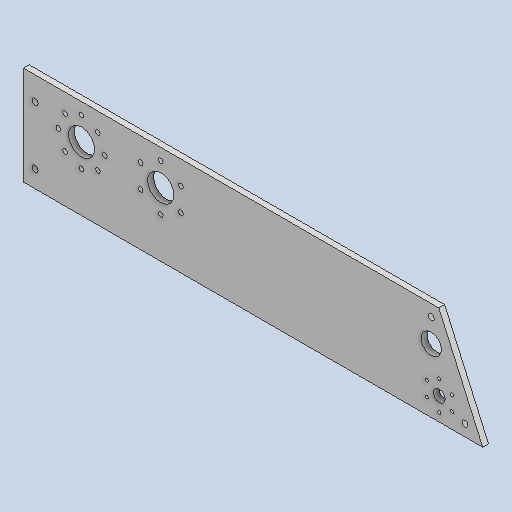
# Autodesk Inventor part: Bottom Part
Saved by Autodesk Inventor 2023 (Build 270158000, 158)
## iProperties
Created: 2023-11-04
Part Number: Bottom Part
Material: Generic
Document SubType Name: Modeling
Designer: jackc
Density: 1 g/cm^3
Appearance: Default
Author: jackc
Autodesk Inventor part; units mm, degrees
ref_plane "YZ Plane" through (0, 0, 0) normal (1, 0, 0) x (0, 1, 0)
ref_plane "XZ Plane" through (0, 0, 0) normal (0, 1, 0) x (-1, 0, 0)
ref_plane "XY Plane" through (0, 0, 0) normal (0, 0, 1) x (1, 0, 0)
sketch "Sketch1" plane through (0, 0, 0) normal (0, 0, 1) x (1, 0, 0)
  circle A0 centre (86.772, 0) radius 50.8 construction
  circle A1 centre (0, 0) radius 29.972 construction
  circle A2 centre (0, 0) radius 25.4 construction
  circle A3 centre (0, 25.4) radius 2.54
  circle A4 centre (17.9605, 17.9605) radius 2.54
  circle A5 centre (-17.9605, 17.9605) radius 2.54
  circle A6 centre (-17.9605, -17.9605) radius 2.54
  circle A7 centre (-25.4, 0) radius 2.54
  circle A8 centre (17.9605, -17.9605) radius 2.54
  circle A9 centre (25.4, 0) radius 2.54
  circle A10 centre (0, -25.4) radius 2.54
  line L0 (0, 25.4) -> (0, 0) construction
  line L1 (0, 0) -> (-17.9605, 17.9605) construction
  circle A11 centre (0, 0) radius 35.972 construction
  line L2 (-63.5, 38.1) -> (-63.5, -69.85)
  line L3 (-63.5, -69.85) -> (438.9497, -69.85)
  circle A12 centre (-50.8, 12.7) radius 3.302
  circle A13 centre (-50.8, -50.8) radius 3.302
  line L4 (-63.5, 38.1) -> (390.9326, 38.1)
  circle A14 centre (86.772, 0) radius 14.2875
  circle A15 centre (0, 0) radius 14.2875
  circle A16 centre (86.772, 0) radius 285.75 construction
  circle A17 centre (382.682, 25.4) radius 3.302
  circle A18 centre (419.4009, -57.15) radius 3.302
  circle A19 centre (86.772, 0) radius 25.4 construction
  circle A20 centre (86.772, 25.4) radius 2.54
  circle A21 centre (64.775, 12.7) radius 2.54
  circle A22 centre (64.775, -12.7) radius 2.54
  circle A23 centre (86.772, -25.4) radius 2.54
  circle A24 centre (108.769, -12.7) radius 2.54
  circle A25 centre (108.769, 12.7) radius 2.54
  circle A26 centre (391.4609, -44.8692) radius 16 construction
  circle A27 centre (391.4609, -44.8692) radius 6.4135
  circle A28 centre (391.4609, -28.8692) radius 1.8
  circle A29 centre (391.4609, -44.8692) radius 22.225 construction
  circle A30 centre (377.6045, -36.8692) radius 1.8
  circle A31 centre (377.6045, -52.8692) radius 1.8
  circle A32 centre (391.4609, -60.8692) radius 1.8
  circle A33 centre (405.3173, -52.8692) radius 1.8
  circle A34 centre (405.3173, -36.8692) radius 1.8
  circle A35 centre (382.682, 0) radius 11.1125
  circle A36 centre (382.682, 0) radius 10.16 construction
  line L5 (438.9497, -69.85) -> (390.9326, 38.1)
  point P0 (328.7742, 38.1)
  point P1 (341.6228, 38.1)
  dimension "d2" = 50.8
  dimension "d32" = 32
  dimension "d0" = 101.6
  dimension "d1" = 59.944
  dimension "d3" = 5.08
  dimension "d4" = 45
  dimension "d5" = 6
  dimension "d6" = 6.604
  dimension "d7" = 63.5
  dimension "d8" = 25.4
  dimension "d9" = 12.7
  dimension "d11" = 19.05
  dimension "d12" = 38.1
  dimension "d13" = 28.575
  dimension "d14" = 28.575
  dimension "d19" = 571.5
  dimension "d30" = 360
  dimension "d33" = 12.827
  dimension "d34" = 3.6
  dimension "d35" = 44.45
  dimension "d38" = 360
  dimension "d40" = 22.225
  dimension "d41" = 20.32
  dimension "d42" = 45.72
  dimension "d43" = 27.94
  dimension "d44" = 50.8
  dimension "d45" = 12.7
  dimension "d46" = 12.7
  dimension "d47" = 12.7
  dimension "d48" = 12.7
  constraints: 34 centre point, 12 end point, 11 equal radius, 10 coincident, 9 vertical alignment, 7 horizontal alignment, 3 tangent, 2 point on line, 2 vertical, 1 concentric, 1 horizontal, 1 perpendicular, 41 other
  measures "d0" diameter of A0
  measures "d1" diameter of A1
  measures "d3" diameter of A5
  measures "d4" angle of L1 L0
  measures "d5" radial gap between concentric circles of A11 A1
  measures "d6" diameter of A12
  measures "d7" distance of A13.centre A12.centre
  measures "d8" horizontal distance of A7.centre A12.centre
  measures "d9" distance from line of L2 A13.centre
  measures "d11" distance from line of A13.centre L3
  measures "d12" distance from line of A11.centre L4
  measures "d13" diameter of A14
  measures "d14" diameter of A15
  measures "d19" diameter of A16
  measures "d33" diameter of A27
  measures "d34" diameter of A28
  measures "d35" diameter of A29
  measures "d40" diameter of A35
  measures "d41" diameter of A36
  measures "d42" distance of point (391.461, -44.869) A35.centre
  measures "d43" horizontal distance of point (391.461, -44.869) A18.centre
  measures "d44" vertical distance of A13.centre A0.centre
  measures "d45" distance from line of A17.centre L4
  measures "d46" distance from line of L3 A18.centre
  measures "d47" distance from line of L5 A17.centre
  measures "d48" distance from line of L5 A18.centre
extrude "Extrusion1" add sketch "Sketch1" along normal blind 6.35
equation "\"WheelSize1\" = 101.6"
body "Solid1"
